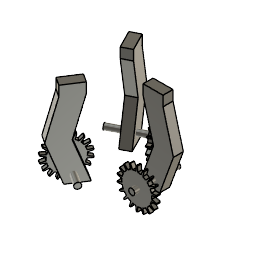
assembly_without_electronics (Autodesk Fusion 360 archive; units mm, degrees)
design "Fingers"
part number: 2026-03-20-16-49-33-089
Autodesk Fusion 360 part; units mm, degrees
sketch "Sketch2" plane through (0, 0, 0) normal (0, 0, 1) x (1, 0, 0)
  circle A0 centre (-139.7, 25.4) radius 19.05
  line L0 (-140.9543, 44.4087) -> (-140.4015, 50.7345)
  line L1 (-138.4228, 44.4071) -> (-138.9798, 50.7327)
  line L2 (-140.4015, 50.7345) -> (-138.9798, 50.7327)
  line L3 (-145.0006, 43.6977) -> (-147.6875, 49.4512)
  line L4 (-149.0241, 48.9668) -> (-147.6875, 49.4512)
  line L5 (-147.38, 42.8333) -> (-149.0241, 48.9668)
  line L6 (-150.9392, 40.7813) -> (-155.4318, 45.2689)
  line L7 (-156.5221, 44.3565) -> (-155.4318, 45.2689)
  line L8 (-152.8794, 39.1552) -> (-156.5221, 44.3565)
  line L9 (-155.5221, 36.0097) -> (-161.2786, 38.69)
  line L10 (-161.9911, 37.4598) -> (-161.2786, 38.69)
  line L11 (-156.7891, 33.8181) -> (-161.9911, 37.4598)
  line L12 (-158.1966, 29.9584) -> (-164.5227, 30.5082)
  line L13 (-164.7715, 29.1085) -> (-164.5227, 30.5082)
  line L14 (-158.6377, 27.4656) -> (-164.7715, 29.1085)
  line L15 (-158.6402, 23.3572) -> (-164.7729, 21.7103)
  line L16 (-164.5279, 20.3099) -> (-164.7729, 21.7103)
  line L17 (-158.2021, 20.8639) -> (-164.5279, 20.3099)
  line L18 (-156.7993, 17.0025) -> (-161.9988, 13.3574)
  line L19 (-161.2896, 12.1252) -> (-161.9988, 13.3574)
  line L20 (-155.5348, 14.8094) -> (-161.2896, 12.1252)
  line L21 (-152.896, 11.6607) -> (-156.5352, 6.457)
  line L22 (-155.4474, 5.5417) -> (-156.5352, 6.457)
  line L23 (-150.9577, 10.0323) -> (-155.4474, 5.5417)
  line L24 (-147.401, 7.976) -> (-149.041, 1.8414)
  line L25 (-147.7058, 1.3534) -> (-149.041, 1.8414)
  line L26 (-145.0227, 7.1087) -> (-147.7058, 1.3534)
  line L27 (-140.9772, 6.3929) -> (-140.4202, 0.0673)
  line L28 (-138.9985, 0.0655) -> (-140.4202, 0.0673)
  line L29 (-138.4457, 6.3913) -> (-138.9985, 0.0655)
  line L30 (-134.3994, 7.1023) -> (-131.7125, 1.3488)
  line L31 (-130.3759, 1.8332) -> (-131.7125, 1.3488)
  line L32 (-132.02, 7.9667) -> (-130.3759, 1.8332)
  line L33 (-128.4608, 10.0187) -> (-123.9682, 5.5311)
  line L34 (-122.8779, 6.4435) -> (-123.9682, 5.5311)
  line L35 (-126.5206, 11.6448) -> (-122.8779, 6.4435)
  line L36 (-123.8779, 14.7903) -> (-118.1214, 12.11)
  line L37 (-117.4089, 13.3402) -> (-118.1214, 12.11)
  line L38 (-122.6109, 16.9819) -> (-117.4089, 13.3402)
  line L39 (-121.2034, 20.8416) -> (-114.8773, 20.2918)
  line L40 (-114.6285, 21.6915) -> (-114.8773, 20.2918)
  line L41 (-120.7623, 23.3344) -> (-114.6285, 21.6915)
  line L42 (-120.7598, 27.4428) -> (-114.6272, 29.0897)
  line L43 (-114.8722, 30.4901) -> (-114.6272, 29.0897)
  line L44 (-121.1979, 29.9361) -> (-114.8722, 30.4901)
  line L45 (-122.6007, 33.7975) -> (-117.4012, 37.4426)
  line L46 (-118.1104, 38.6748) -> (-117.4012, 37.4426)
  line L47 (-123.8652, 35.9906) -> (-118.1104, 38.6748)
  line L48 (-126.5041, 39.1393) -> (-122.8648, 44.343)
  line L49 (-123.9526, 45.2583) -> (-122.8648, 44.343)
  line L50 (-128.4423, 40.7677) -> (-123.9526, 45.2583)
  line L51 (-131.999, 42.824) -> (-130.359, 48.9586)
  line L52 (-131.6942, 49.4466) -> (-130.359, 48.9586)
  line L53 (-134.3773, 43.6913) -> (-131.6942, 49.4466)
  dimension "d14" = 38.1
  dimension "d15" = 6.35
  dimension "d16" = 6.35
  dimension "d18" = 360
  constraint coincident A0 L0.start
  constraint coincident A0 L1.start
  measures "d14" diameter of A0
  measures "d15" distance of L0.start L0.end
  measures "d16" distance of L1.start L1.end
extrude "Extrude3" add sketch "Sketch2" along normal blind 5.08 makes body 1
sketch "Sketch3" plane through (0, 0, 0) normal (0, 0, 1) x (1, 0, 0)
  line L0 (0, 0) -> (17.3334, 47.7514)
  line L1 (-25.4, 0) -> (-7.9907, 47.7237)
  line L2 (17.3334, 47.7514) -> (4.2196, 96.8296)
  line L3 (-7.9907, 47.7237) -> (-21.1192, 96.798)
  line L4 (-21.1192, 96.798) -> (4.2196, 96.8296)
  line L5 (-25.4, 0) -> (0, 0)
  dimension "d21" = 50.8
  dimension "d22" = 50.8
  dimension "d23" = 50.8
  dimension "d24" = 50.8
  constraint coincident L0.start L5.end
  constraint horizontal L5
  measures "d21" distance of L0.start L0.end
  measures "d22" distance of L1.start L1.end
  measures "d23" distance of L0.end L2.end
  measures "d24" distance of L1.end L3.end
extrude "Extrude4" add sketch "Sketch3" along normal blind 12.7 separate body makes body 2
move_body "Move2" bodies 1 to x (1, 0, 0) y (0, 1, 0) z (0, 0, 1) at (130.81, -15.24, 12.7)
sketch "Sketch4" plane through (0, 0, 17.78) normal (0, 0, 1) x (-1, 0, 0)
  line L0 (7.6128, -29.1671) -> (8.1698, -35.4927)
  line L1 (8.1698, -35.4927) -> (9.5915, -35.4945)
  line L2 (9.5915, -35.4945) -> (10.1443, -29.1687)
  arc A0 (10.1443, -29.1687) -> (14.1906, -28.4577) centre (8.89, -10.16) ccw
  line L3 (14.1906, -28.4577) -> (16.8775, -34.2112)
  line L4 (16.8775, -34.2112) -> (18.2141, -33.7268)
  line L5 (18.2141, -33.7268) -> (16.57, -27.5933)
  arc A1 (16.57, -27.5933) -> (20.1292, -25.5413) centre (8.89, -10.16) ccw
  line L6 (20.1292, -25.5413) -> (24.6218, -30.0289)
  line L7 (24.6218, -30.0289) -> (25.7121, -29.1165)
  line L8 (25.7121, -29.1165) -> (22.0694, -23.9152)
  arc A2 (22.0694, -23.9152) -> (24.7121, -20.7697) centre (8.89, -10.16) ccw
  line L9 (24.7121, -20.7697) -> (30.4686, -23.45)
  line L10 (30.4686, -23.45) -> (31.1811, -22.2198)
  line L11 (31.1811, -22.2198) -> (25.9791, -18.5781)
  arc A3 (25.9791, -18.5781) -> (27.3866, -14.7184) centre (8.89, -10.16) ccw
  line L12 (27.3866, -14.7184) -> (33.7127, -15.2682)
  line L13 (33.7127, -15.2682) -> (33.9615, -13.8685)
  line L14 (33.9615, -13.8685) -> (27.8277, -12.2256)
  arc A4 (27.8277, -12.2256) -> (27.8302, -8.1172) centre (8.89, -10.16) ccw
  line L15 (27.8302, -8.1172) -> (33.9629, -6.4703)
  line L16 (33.9629, -6.4703) -> (33.7179, -5.0699)
  line L17 (33.7179, -5.0699) -> (27.3921, -5.6239)
  arc A5 (27.3921, -5.6239) -> (25.9893, -1.7625) centre (8.89, -10.16) ccw
  line L18 (25.9893, -1.7625) -> (31.1888, 1.8826)
  line L19 (31.1888, 1.8826) -> (30.4796, 3.1148)
  line L20 (30.4796, 3.1148) -> (24.7248, 0.4306)
  arc A6 (24.7248, 0.4306) -> (22.086, 3.5793) centre (8.89, -10.16) ccw
  line L21 (22.086, 3.5793) -> (25.7252, 8.783)
  line L22 (25.7252, 8.783) -> (24.6374, 9.6983)
  line L23 (24.6374, 9.6983) -> (20.1477, 5.2077)
  arc A7 (20.1477, 5.2077) -> (16.591, 7.264) centre (8.89, -10.16) ccw
  line L24 (16.591, 7.264) -> (18.231, 13.3986)
  line L25 (18.231, 13.3986) -> (16.8958, 13.8866)
  line L26 (16.8958, 13.8866) -> (14.2127, 8.1313)
  arc A8 (14.2127, 8.1313) -> (10.1672, 8.8471) centre (8.89, -10.16) ccw
  line L27 (10.1672, 8.8471) -> (9.6102, 15.1727)
  line L28 (9.6102, 15.1727) -> (8.1885, 15.1745)
  line L29 (8.1885, 15.1745) -> (7.6357, 8.8487)
  arc A9 (7.6357, 8.8487) -> (3.5894, 8.1377) centre (8.89, -10.16) ccw
  line L30 (3.5894, 8.1377) -> (0.9025, 13.8912)
  line L31 (0.9025, 13.8912) -> (-0.4341, 13.4068)
  line L32 (-0.4341, 13.4068) -> (1.21, 7.2733)
  arc A10 (1.21, 7.2733) -> (-2.3492, 5.2213) centre (8.89, -10.16) ccw
  line L33 (-2.3492, 5.2213) -> (-6.8418, 9.7089)
  line L34 (-6.8418, 9.7089) -> (-7.9321, 8.7965)
  line L35 (-7.9321, 8.7965) -> (-4.2894, 3.5952)
  arc A11 (-4.2894, 3.5952) -> (-6.9321, 0.4497) centre (8.89, -10.16) ccw
  line L36 (-6.9321, 0.4497) -> (-12.6886, 3.13)
  line L37 (-12.6886, 3.13) -> (-13.4011, 1.8998)
  line L38 (-13.4011, 1.8998) -> (-8.1991, -1.7419)
  arc A12 (-8.1991, -1.7419) -> (-9.6066, -5.6016) centre (8.89, -10.16) ccw
  line L39 (-9.6066, -5.6016) -> (-15.9327, -5.0518)
  line L40 (-15.9327, -5.0518) -> (-16.1815, -6.4515)
  line L41 (-16.1815, -6.4515) -> (-10.0477, -8.0944)
  arc A13 (-10.0477, -8.0944) -> (-10.0502, -12.2028) centre (8.89, -10.16) ccw
  line L42 (-10.0502, -12.2028) -> (-16.1828, -13.8497)
  line L43 (-16.1828, -13.8497) -> (-15.9378, -15.2501)
  line L44 (-15.9378, -15.2501) -> (-9.6121, -14.6961)
  arc A14 (-9.6121, -14.6961) -> (-8.2093, -18.5575) centre (8.89, -10.16) ccw
  line L45 (-8.2093, -18.5575) -> (-13.4088, -22.2026)
  line L46 (-13.4088, -22.2026) -> (-12.6996, -23.4348)
  line L47 (-12.6996, -23.4348) -> (-6.9448, -20.7506)
  arc A15 (-6.9448, -20.7506) -> (-4.3059, -23.8993) centre (8.89, -10.16) ccw
  line L48 (-4.3059, -23.8993) -> (-7.9452, -29.103)
  line L49 (-7.9452, -29.103) -> (-6.8574, -30.0183)
  line L50 (-6.8574, -30.0183) -> (-2.3677, -25.5277)
  arc A16 (-2.3677, -25.5277) -> (1.189, -27.584) centre (8.89, -10.16) ccw
  line L51 (1.189, -27.584) -> (-0.451, -33.7186)
  line L52 (-0.451, -33.7186) -> (0.8842, -34.2066)
  line L53 (0.8842, -34.2066) -> (3.5673, -28.4513)
  arc A17 (3.5673, -28.4513) -> (7.6128, -29.1671) centre (8.89, -10.16) ccw
  circle A18 centre (8.89, -10.16) radius 3.81
  dimension "d27" = 7.62
  constraint concentric A0 A18
  measures "d27" diameter of A18
extrude "Extrude5" add sketch "Sketch4" along normal mid plane 58.42 separate body contours A18 makes body 3
move_body "Move3" bodies 3 to x (1, 0, 0) y (0, 1, 0) z (0, 0, 1) at (0, 0, -7.62)
copy_body "CopyPasteBodies1" bodies 2 makes body 4
move_body "Move4" bodies 4 to x (1, 0, 0) y (0, 1, 0) z (0, 0, 1) at (-88.9, 0, 0)
copy_body "CopyPasteBodies2" bodies 3 makes body 5
move_body "Move5" bodies 5 to x (1, 0, 0) y (0, 1, 0) z (0, 0, 1) at (-88.9, 0, 0)
copy_body "CopyPasteBodies3" bodies 1 makes body 6
move_body "Move6" bodies 6 to x (1, 0, 0) y (0, 1, 0) z (0, 0, 1) at (-88.9, 0, 0)
copy_body "CopyPasteBodies4" bodies 4 6 5 makes body 7 makes body 8 makes body 9
move_body "Move7" bodies 7 8 9 to x (1, 0, 0) y (0, 1, 0) z (0, 0, 1) at (-88.9, 0, 0)
move_body "Move8" bodies 7 9 8 to x (1, 0, 0) y (0, 0, 1) z (0, -1, 0) at (0, 61.1148, -35.7148)
move_body "Move9" bodies 4 6 5 to x (1, 0, 0) y (0, 0, 1) z (0, -1, 0) at (0, 61.1148, -35.7148)
move_body "Move10" bodies 2 1 3 to x (1, 0, 0) y (0, 0, 1) z (0, -1, 0) at (0, 61.1148, -35.7148)
move_body "Move12" bodies 7 9 8 to x (-0.499998, -0.866025, -0.001867) y (0.866025, -0.5, 0.001078) z (-0.001867, -0.001078, 0.999998) at (-232.0022, -105.7721, 54.0724)
move_body "Move13" bodies 2 3 1 to x (1, 0, 0) y (0, 1, 0) z (0, 0, 1) at (13.057, 0, 35.7928)
move_body "Move14" bodies 7 8 9 to x (1, 0, 0) y (0, 1, 0) z (0, 0, 1) at (0.0119, -0.0068, -12.7)
move_body "Move15" bodies 4 5 6 to x (-0.499998, 0.866025, -0.001867) y (-0.866025, -0.5, -0.001078) z (-0.001867, 0.001078, 0.999998) at (-79.3477, 216.7581, 35.0807)
move_body "Move16" bodies 7 9 8 to x (0.996195, 0.087156, -0.000005) y (-0.087156, 0.996195, -0.000108) z (-0.000005, 0.000108, 1) at (52.7816, -0.8822, 0.0657)
move_body "Move17" bodies 4 5 6 to x (1, 0, 0) y (0, 1, 0) z (0, 0, 1) at (35.5478, -23.4706, 0.0443)
move_body "Move18" bodies 7 9 8 to x (1, 0, 0) y (0, 1, 0) z (0, 0, 1) at (0, 6.35, 0)
move_body "Move19" bodies 7 9 8 to x (0.996195, -0.087156, -0.000005) y (0.087156, 0.996195, 0.000108) z (-0.000005, -0.000108, 1) at (-2.3742, -3.4539, -0.003)
move_body "Move20" bodies 7 8 9 to x (1, 0, 0) y (0, 1, 0) z (0, 0, 1) at (-5.08, -5.08, -0.0063)
move_body "Move21" bodies 7 8 9 to x (0.996195, 0.087156, -0.000005) y (-0.087156, 0.996195, -0.000108) z (-0.000005, 0.000108, 1) at (-3.4779, -1.0089, -0.0043)
move_body "Move22" bodies 7 8 9 to x (0.984808, -0.173648, -0.000019) y (0.173648, 0.984808, 0.000216) z (-0.000019, -0.000216, 1) at (-8.5106, -13.6864, -0.0106)
move_body "Move23" bodies 7 8 9 to x (1, 0, 0) y (0, 1, 0) z (0, 0, 1) at (-5.08, -5.08, -0.0063)
move_body "Move24" bodies 7 9 8 to x (1, 0, 0) y (0, 1, 0) z (0, 0, 1) at (2.54, 2.54, 0.0032)
move_body "Move25" bodies 7 8 9 to x (1, 0, 0) y (0, 1, 0) z (0, 0, 1) at (0.0053, -0.0037, -6.35)
move_body "Move26" bodies 4 5 6 to x (1, 0, 0) y (0, 1, 0) z (0, 0, 1) at (-20.32, 20.32, -0.0253)
move_body "Move27" bodies 4 5 6 to x (1, 0, 0) y (0, 1, 0) z (0, 0, 1) at (2.54, -5.08, 0.0032)
move_body "Move28" bodies 4 5 6 to x (1, 0, 0) y (0, 1, 0) z (0, 0, 1) at (-5.08, -5.08, -0.0063)
move_body "Move29" bodies 4 5 6 to x (0.99863, -0.052336, -0.000002) y (0.052336, 0.99863, 0.000065) z (-0.000002, -0.000065, 1) at (-4.8953, -3.2973, -0.0061)
move_body "Move30" bodies 4 5 6 to x (1, 0, 0) y (0, 1, 0) z (0, 0, 1) at (1.1152, -2.1872, -0.6512)
move_body "Move31" bodies 1 to x (1, 0, 0) y (0, 1, 0) z (0, 0, 1) at (0, -15.24, 0)
move_body "Move32" bodies 8 to x (1, 0, 0) y (0, 1, 0) z (0, 0, 1) at (-12.4839, 8.7413, -0.0155)
move_body "Move33" bodies 6 to x (1, 0, 0) y (0, 1, 0) z (0, 0, 1) at (13.5789, 6.9188, 0.0169)
extrude "Extrude6" add 1 faces at (0.3841, 52.6481, 96.8866) along direction (-0.001245, 0, 0.999999) blind 12.7 on bodies 2 bodies 2
extrude "Extrude7" add 1 faces at (-54.4878, 9.9242, 96.5742) along direction (-0.001245, 0, 0.999999) blind 12.7 on bodies 7 bodies 7
extrude "Extrude8" add 1 faces at (-60.6085, 86.8346, 95.6716) along direction (-0.001245, 0, 0.999999) blind 12.7 on bodies 4 bodies 4
move_body "Move34" bodies 7 9 8 to x (0.996195, 0.087156, -0.000005) y (-0.087156, 0.996195, -0.000108) z (-0.000005, 0.000108, 1) at (0.4466, 5.1299, 0.0006)
move_body "Move35" bodies 7 9 8 to x (0.99863, -0.052336, -0.000002) y (0.052336, 0.99863, 0.000065) z (-0.000002, -0.000065, 1) at (-0.4821, -3.0524, -0.0006)

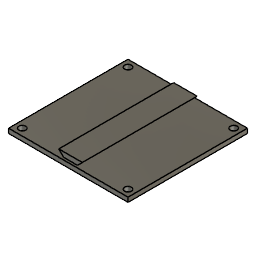
design "base_bottom"
part number: 2026-03-16-14-32-38-053
Autodesk Fusion 360 part; units mm, degrees
sketch "Sketch5" plane through (0, 0, 0) normal (0, 0, 1) x (1, 0, 0)
  line L0 (66.04, -66.04) -> (-66.04, -66.04)
  line L1 (-66.04, -66.04) -> (-66.04, 66.04)
  line L2 (-66.04, 66.04) -> (66.04, 66.04)
  line L3 (66.04, 66.04) -> (66.04, -66.04)
  line L4 (66.04, -66.04) -> (-66.04, 66.04) construction
  line L5 (-66.04, -66.04) -> (66.04, 66.04) construction
  constraint horizontal L0
  constraint perpendicular L0 L1
  constraint parallel L0 L2
  constraint parallel L1 L3
  constraint coincident L4 origin
  constraint coincident L5 origin
extrude "Extrude8" add sketch "Sketch5" along normal blind 5.08 makes body 1
sketch "Sketch6" plane through (0, 0, 5.08) normal (0, 0, 1) x (-1, 0, 0)
  line L0 (-66.04, -66.04) -> (66.04, -66.04)
  line L1 (66.04, -66.04) -> (66.04, 66.04)
  line L2 (66.04, 66.04) -> (-66.04, 66.04)
  line L3 (-66.04, 66.04) -> (-66.04, -66.04)
  circle A0 centre (58.42, -58.42) radius 3.81
  circle A1 centre (-58.42, -58.42) radius 3.81
  circle A2 centre (58.42, 58.42) radius 3.81
  circle A3 centre (-58.42, 58.42) radius 3.81
  dimension "d26" = 7.62
  dimension "d27" = 7.62
  dimension "d28" = 7.62
  dimension "d29" = 7.62
  measures "d26" diameter of A0
  measures "d27" diameter of A1
  measures "d28" diameter of A2
  measures "d29" diameter of A3
extrude "Extrude9" cut sketch "Sketch6" against normal blind 15.24 contours A0 | A1 | A2 | A3 bodies 1
sketch "Sketch7" plane through (0, 0, 5.08) normal (0, 0, 1) x (-1, 0, 0)
  circle A0 centre (58.42, -58.42) radius 3.81
  circle A1 centre (-58.42, -58.42) radius 3.81
  circle A2 centre (58.42, 58.42) radius 3.81
  circle A3 centre (-58.42, 58.42) radius 3.81
  line L0 (-66.04, -66.04) -> (66.04, -66.04)
  line L1 (66.04, -66.04) -> (66.04, 66.04)
  line L2 (66.04, 66.04) -> (-66.04, 66.04)
  line L3 (-66.04, 66.04) -> (-66.04, -66.04)
  circle A4 centre (0, 0) radius 62.8904
  dimension "d32" = 125.7808
  constraint coincident A4.centre origin
  measures "d32" diameter of A4
sketch "Sketch8" plane through (0, 0, 0) normal (0, 1, 0) x (1, 0, 0)
  line L0 (-7.62, -7.62) -> (-13.006, -13.0103)
  line L1 (7.62, -7.62) -> (13.0103, -13.006)
  line L2 (13.0103, -13.006) -> (-13.006, -13.0103)
  line L3 (7.62, -7.62) -> (-7.62, -7.62)
  dimension "d35" = 7.62
  dimension "d36" = 7.62
  constraint perpendicular L0 L1
  constraint horizontal L3
  measures "d35" distance of L0.start L0.end
  measures "d36" distance of L1.start L1.end
extrude "Extrude11" add sketch "Sketch8" along normal blind 63.5 and the other way blind 63.5 separate body makes body 2
move_body "Move1" bodies 2 to x (1, 0, 0) y (0, 1, 0) z (0, 0, 1) at (-0.0004, 0, -2.54)

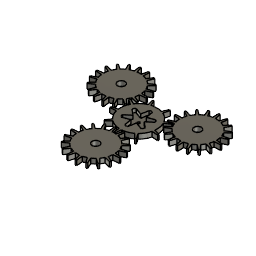
design "finger_gears" references "arm_middle"
part number: 2026-03-18-13-44-59-232
Autodesk Fusion 360 part; units mm, degrees
other "ExternalDerived1"
sketch "Sketch7" plane through (0, 0, 0) normal (0, 0, 1) x (1, 0, 0)
  circle A0 centre (0, 0) radius 19.05
  line L0 (1.2658, -19.0079) -> (0.716, -25.3341)
  line L1 (-1.3142, -19.0046) -> (-0.7583, -25.3302)
  line L2 (0.716, -25.3341) -> (-0.7583, -25.3302)
  line L3 (7.6905, -17.4287) -> (9.3375, -23.5613)
  line L4 (9.3375, -23.5613) -> (7.9509, -24.062)
  line L5 (5.265, -18.308) -> (7.9509, -24.062)
  line L6 (13.1877, -13.7473) -> (16.8329, -18.9468)
  line L7 (16.8329, -18.9468) -> (15.7011, -19.8915)
  line L8 (11.2092, -15.4031) -> (15.7011, -19.8915)
  line L9 (17.0942, -8.4078) -> (22.2979, -12.047)
  line L10 (22.2979, -12.047) -> (21.5575, -13.3218)
  line L11 (15.8014, -10.6405) -> (21.5575, -13.3218)
  line L12 (18.9389, -2.0541) -> (25.0735, -3.6941)
  line L13 (25.0735, -3.6941) -> (24.8137, -5.1453)
  line L14 (18.4877, -4.5944) -> (24.8137, -5.1453)
  line L15 (18.4993, 4.5472) -> (24.8248, 5.1043)
  line L16 (24.8248, 5.1043) -> (25.0771, 3.6518)
  line L17 (18.9441, 2.0059) -> (25.0771, 3.6518)
  line L18 (15.8284, 10.6001) -> (21.582, 13.2871)
  line L19 (21.582, 13.2871) -> (22.3158, 12.0084)
  line L20 (17.1156, 8.3642) -> (22.3158, 12.0084)
  line L21 (11.2484, 15.3745) -> (15.736, 19.8672)
  line L22 (15.736, 19.8672) -> (16.8628, 18.9167)
  line L23 (13.2227, 13.7136) -> (16.8628, 18.9167)
  line L24 (5.3116, 18.2945) -> (7.992, 24.0511)
  line L25 (7.992, 24.0511) -> (9.376, 23.5433)
  line L26 (7.7349, 17.409) -> (9.376, 23.5433)
  line L27 (-1.2658, 19.0079) -> (-0.716, 25.3341)
  line L28 (-0.716, 25.3341) -> (0.7583, 25.3302)
  line L29 (1.3142, 19.0046) -> (0.7583, 25.3302)
  line L30 (-7.6905, 17.4287) -> (-9.3375, 23.5613)
  line L31 (-9.3375, 23.5613) -> (-7.9509, 24.062)
  line L32 (-5.265, 18.308) -> (-7.9509, 24.062)
  line L33 (-13.1877, 13.7473) -> (-16.8329, 18.9468)
  line L34 (-16.8329, 18.9468) -> (-15.7011, 19.8915)
  line L35 (-11.2092, 15.4031) -> (-15.7011, 19.8915)
  line L36 (-17.0942, 8.4078) -> (-22.2979, 12.047)
  line L37 (-22.2979, 12.047) -> (-21.5575, 13.3218)
  line L38 (-15.8014, 10.6405) -> (-21.5575, 13.3218)
  line L39 (-18.9389, 2.0541) -> (-25.0735, 3.6941)
  line L40 (-25.0735, 3.6941) -> (-24.8137, 5.1453)
  line L41 (-18.4877, 4.5944) -> (-24.8137, 5.1453)
  line L42 (-18.4993, -4.5472) -> (-24.8248, -5.1043)
  line L43 (-24.8248, -5.1043) -> (-25.0771, -3.6518)
  line L44 (-18.9441, -2.0059) -> (-25.0771, -3.6518)
  line L45 (-15.8284, -10.6001) -> (-21.582, -13.2871)
  line L46 (-21.582, -13.2871) -> (-22.3158, -12.0084)
  line L47 (-17.1156, -8.3642) -> (-22.3158, -12.0084)
  line L48 (-11.2484, -15.3745) -> (-15.736, -19.8672)
  line L49 (-15.736, -19.8672) -> (-16.8628, -18.9167)
  line L50 (-13.2227, -13.7136) -> (-16.8628, -18.9167)
  line L51 (-5.3116, -18.2945) -> (-7.992, -24.0511)
  line L52 (-7.992, -24.0511) -> (-9.376, -23.5433)
  line L53 (-7.7349, -17.409) -> (-9.376, -23.5433)
  dimension "d61" = 38.1
  dimension "d62" = 6.35
  dimension "d63" = 6.35
  dimension "d65" = 360
  constraint coincident A0.centre origin
  constraint coincident A0 L0.start
  constraint coincident A0 L1.start
  measures "d61" diameter of A0
  measures "d62" distance of L0.start L0.end
  measures "d63" distance of L1.start L1.end
extrude "Extrude7" add sketch "Sketch7" along normal blind 5.08 makes body 1
copy_body "CopyPasteBodies1" bodies 1 makes body 2
move_body "Move19" bodies 2 to x (1, 0, 0) y (0, 1, 0) z (0, 0, 1) at (-60.96, 0, 0)
copy_body "CopyPasteBodies2" bodies 1 makes body 3
move_body "Move20" bodies 3 to x (1, 0, 0) y (0, 1, 0) z (0, 0, 1) at (73.66, 0, 0)
sketch "Sketch8" plane through (0, 0, 0) normal (0, 0, 1) x (1, 0, 0)
  circle A0 centre (0, 76.2) radius 19.05
  line L0 (1.2378, 57.1903) -> (0.685, 50.8644)
  line L1 (-1.2378, 57.1903) -> (-0.6861, 50.8643)
  line L2 (0.685, 50.8644) -> (-0.6861, 50.8643)
  line L3 (16.8102, 57.2321) -> (15.7599, 56.3507)
  line L4 (13.1674, 62.4333) -> (16.8102, 57.2321)
  line L5 (11.271, 60.842) -> (15.7599, 56.3507)
  line L6 (25.0697, 72.4751) -> (24.8317, 71.1248)
  line L7 (18.9359, 74.118) -> (25.0697, 72.4751)
  line L8 (18.506, 71.68) -> (24.8317, 71.1248)
  line L9 (21.5988, 89.4611) -> (22.2844, 88.2737)
  line L10 (15.844, 86.7769) -> (21.5988, 89.4611)
  line L11 (17.0818, 84.6329) -> (22.2844, 88.2737)
  line L12 (8.0216, 100.242) -> (9.31, 99.7731)
  line L13 (5.3385, 94.4867) -> (8.0216, 100.242)
  line L14 (7.6649, 93.64) -> (9.31, 99.7731)
  line L15 (-9.309, 99.7734) -> (-8.0206, 100.2425)
  line L16 (-7.6649, 93.64) -> (-9.309, 99.7734)
  line L17 (-5.3385, 94.4867) -> (-8.0206, 100.2425)
  line L18 (-22.2838, 88.2746) -> (-21.5983, 89.462)
  line L19 (-17.0818, 84.6329) -> (-22.2838, 88.2746)
  line L20 (-15.844, 86.7769) -> (-21.5983, 89.462)
  line L21 (-24.8318, 71.1259) -> (-25.07, 72.4762)
  line L22 (-18.506, 71.68) -> (-24.8318, 71.1259)
  line L23 (-18.9359, 74.118) -> (-25.07, 72.4762)
  line L24 (-15.7607, 56.3514) -> (-16.8111, 57.2327)
  line L25 (-11.271, 60.842) -> (-15.7607, 56.3514)
  line L26 (-13.1674, 62.4333) -> (-16.8111, 57.2327)
  dimension "d68" = 38.1
  dimension "d69" = 6.35
  dimension "d70" = 6.35
  dimension "d72" = 360
  constraint coincident A0 L0.start
  constraint coincident A0 L1.start
  measures "d68" diameter of A0
  measures "d69" distance of L0.start L0.end
  measures "d70" distance of L1.start L1.end
extrude "Extrude8" add sketch "Sketch8" along normal blind 5.08 separate body makes body 4
move_body "Move21" bodies 4 to x (1, 0, 0) y (0, 1, 0) z (0, 0, 1) at (43.18, -38.1, 0)
move_body "Move22" bodies 4 to x (1, 0, 0) y (0, 1, 0) z (0, 0, 1) at (-5.08, 0, 0)
move_body "Move23" bodies 4 to x (-1, 0, 0) y (0, 1, 0) z (0, 0, -1) at (76.2, 0, 7.62)
move_body "Move24" bodies 3 to x (0.990268, -0.139173, 0) y (0.139173, 0.990268, 0) z (0, 0, 1) at (3.1462, 72.4863, 0)
move_body "Move25" bodies 1 to x (0.999391, 0.034899, 0) y (-0.034899, 0.999391, 0) z (0, 0, 1) at (1.0397, 64.1158, 0.0186)
move_body "Move26" bodies 3 to x (0.965926, -0.258819, 0) y (0.258819, 0.965926, 0) z (0, 0, 1) at (-10.4016, 16.6906, 0.0245)
move_body "Move27" bodies 1 to x (0.939693, 0.34202, 0) y (-0.34202, 0.939693, 0) z (0, 0, 1) at (18.0551, -3.2469, 0.0176)
move_body "Move28" bodies 2 to x (0.984808, -0.173648, 0) y (0.173648, 0.984808, 0) z (0, 0, 1) at (98.3264, -16.9924, 91.5036)
sketch "Sketch13" plane through (0, 0, 96.5836) normal (0, 0, 1) x (-1, 0, 0)
  arc A0 (-24.5452, 19.5945) -> (-27.652, 22.2082) centre (-38.2925, 6.4068) ccw
  line L0 (-27.652, 22.2082) -> (-24.9707, 27.9643)
  line L1 (-24.9707, 27.9643) -> (-26.2455, 28.7047)
  line L2 (-26.2455, 28.7047) -> (-29.8847, 23.501)
  arc A1 (-29.8847, 23.501) -> (-33.6981, 24.8945) centre (-38.2925, 6.4068) ccw
  line L3 (-33.6981, 24.8945) -> (-33.1472, 31.2205)
  line L4 (-33.1472, 31.2205) -> (-34.5984, 31.4803)
  line L5 (-34.5984, 31.4803) -> (-36.2383, 25.3457)
  arc A2 (-36.2383, 25.3457) -> (-40.2983, 25.3509) centre (-38.2925, 6.4068) ccw
  line L6 (-40.2983, 25.3509) -> (-41.9443, 31.4839)
  line L7 (-41.9443, 31.4839) -> (-43.3968, 31.2317)
  line L8 (-43.3968, 31.2317) -> (-42.8397, 24.9061)
  arc A3 (-42.8397, 24.9061) -> (-46.6566, 23.5224) centre (-38.2925, 6.4068) ccw
  line L9 (-46.6566, 23.5224) -> (-50.3009, 28.7226)
  line L10 (-50.3009, 28.7226) -> (-51.5796, 27.9888)
  line L11 (-51.5796, 27.9888) -> (-48.8926, 22.2353)
  arc A4 (-48.8926, 22.2353) -> (-52.0061, 19.6295) centre (-38.2925, 6.4068) ccw
  line L12 (-52.0061, 19.6295) -> (-57.2091, 23.2697)
  line L13 (-57.2091, 23.2697) -> (-58.1597, 22.1428)
  line L14 (-58.1597, 22.1428) -> (-53.667, 17.6552)
  arc A5 (-53.667, 17.6552) -> (-55.7015, 14.1417) centre (-38.2925, 6.4068) ccw
  line L15 (-55.7015, 14.1417) -> (-61.8358, 15.7828)
  line L16 (-61.8358, 15.7828) -> (-62.3436, 14.3988)
  line L17 (-62.3436, 14.3988) -> (-56.587, 11.7185)
  arc A6 (-56.587, 11.7185) -> (-57.2971, 7.721) centre (-38.2925, 6.4068) ccw
  line L18 (-57.2971, 7.721) -> (-63.6227, 7.1651)
  line L19 (-63.6227, 7.1651) -> (-63.6265, 5.6908)
  line L20 (-63.6265, 5.6908) -> (-57.3004, 5.141)
  arc A7 (-57.3004, 5.141) -> (-56.6005, 1.1418) centre (-38.2925, 6.4068) ccw
  line L21 (-56.6005, 1.1418) -> (-62.3545, -1.5441)
  line L22 (-62.3545, -1.5441) -> (-61.8538, -2.9307)
  line L23 (-61.8538, -2.9307) -> (-55.7212, -1.2837)
  arc A8 (-55.7212, -1.2837) -> (-53.6956, -4.8024) centre (-38.2925, 6.4068) ccw
  line L24 (-53.6956, -4.8024) -> (-58.184, -9.2943)
  line L25 (-58.184, -9.2943) -> (-57.2393, -10.4261)
  line L26 (-57.2393, -10.4261) -> (-52.0398, -6.7809)
  arc A9 (-52.0398, -6.7809) -> (-48.9329, -9.3946) centre (-38.2925, 6.4068) ccw
  line L27 (-48.9329, -9.3946) -> (-51.6143, -15.1507)
  line L28 (-51.6143, -15.1507) -> (-50.3395, -15.8911)
  line L29 (-50.3395, -15.8911) -> (-46.7002, -10.6874)
  arc A10 (-46.7002, -10.6874) -> (-42.8869, -12.0809) centre (-38.2925, 6.4068) ccw
  line L30 (-42.8869, -12.0809) -> (-43.4378, -18.4069)
  line L31 (-43.4378, -18.4069) -> (-41.9866, -18.6667)
  line L32 (-41.9866, -18.6667) -> (-40.3466, -12.5321)
  arc A11 (-40.3466, -12.5321) -> (-36.2866, -12.5373) centre (-38.2925, 6.4068) ccw
  line L33 (-36.2866, -12.5373) -> (-34.6407, -18.6703)
  line L34 (-34.6407, -18.6703) -> (-33.1882, -18.418)
  line L35 (-33.1882, -18.418) -> (-33.7453, -12.0925)
  arc A12 (-33.7453, -12.0925) -> (-29.9283, -10.7088) centre (-38.2925, 6.4068) ccw
  line L36 (-29.9283, -10.7088) -> (-26.2841, -15.909)
  line L37 (-26.2841, -15.909) -> (-25.0054, -15.1751)
  line L38 (-25.0054, -15.1751) -> (-27.6923, -9.4216)
  arc A13 (-27.6923, -9.4216) -> (-24.5789, -6.8159) centre (-38.2925, 6.4068) ccw
  line L39 (-24.5789, -6.8159) -> (-19.3758, -10.456)
  line L40 (-19.3758, -10.456) -> (-18.4253, -9.3291)
  line L41 (-18.4253, -9.3291) -> (-22.918, -4.8416)
  arc A14 (-22.918, -4.8416) -> (-20.8835, -1.3281) centre (-38.2925, 6.4068) ccw
  line L42 (-20.8835, -1.3281) -> (-14.7492, -2.9692)
  line L43 (-14.7492, -2.9692) -> (-14.2414, -1.5852)
  line L44 (-14.2414, -1.5852) -> (-19.998, 1.0952)
  arc A15 (-19.998, 1.0952) -> (-19.2879, 5.0926) centre (-38.2925, 6.4068) ccw
  line L45 (-19.2879, 5.0926) -> (-12.9623, 5.6485)
  line L46 (-12.9623, 5.6485) -> (-12.9584, 7.1228)
  line L47 (-12.9584, 7.1228) -> (-19.2846, 7.6726)
  arc A16 (-19.2846, 7.6726) -> (-19.9845, 11.6718) centre (-38.2925, 6.4068) ccw
  line L48 (-19.9845, 11.6718) -> (-14.2305, 14.3577)
  line L49 (-14.2305, 14.3577) -> (-14.7311, 15.7444)
  line L50 (-14.7311, 15.7444) -> (-20.8638, 14.0973)
  arc A17 (-20.8638, 14.0973) -> (-22.8893, 17.616) centre (-38.2925, 6.4068) ccw
  line L51 (-22.8893, 17.616) -> (-18.401, 22.1079)
  line L52 (-18.401, 22.1079) -> (-19.3457, 23.2397)
  line L53 (-19.3457, 23.2397) -> (-24.5452, 19.5945)
  circle A18 centre (-38.2925, 6.4068) radius 3.81
  circle A19 centre (-78.74, -57.15) radius 3.81
  circle A20 centre (3.3176, -57.4165) radius 3.81
  dimension "d93" = 7.62
  dimension "d94" = 7.62
  dimension "d95" = 7.62
  constraint concentric A0 A18
  measures "d93" diameter of A18
  measures "d94" diameter of A19
  measures "d95" diameter of A20
move_body "Move29" bodies 2 to x (1, 0, 0) y (0, 1, 0) z (0, 0, 1) at (0, 0, -88.9)
move_body "Move30" bodies 4 to x (1, 0, 0) y (0, 1, 0) z (0, 0, 1) at (0, 0, -2.54)
move_body "Move31" bodies 2 to x (1, 0, 0) y (0, 1, 0) z (0, 0, 1) at (0, 0, -2.54)
extrude "Extrude11" cut sketch "Sketch13" along normal blind 0 and the other way blind 106.68 contours A18 | A19 | A20 bodies 1 2 3
move_body "Move32" bodies 3 to x (0.984808, -0.173648, 0) y (0.173648, 0.984808, 0) z (0, 0, 1) at (-6.403, 10.7814, -0.0115)
move_body "Move33" bodies 1 to x (0.984808, 0.173648, 0) y (-0.173648, 0.984808, 0) z (0, 0, 1) at (7.6575, -2.701, -0.0412)
move_body "Move34" bodies 3 to x (0.939693, 0.34202, 0) y (-0.34202, 0.939693, 0) z (0, 0, 1) at (20.3537, -18.1148, -0.6132)
move_body "Move35" bodies 1 to x (0.939693, -0.34202, 0) y (0.34202, 0.939693, 0) z (0, 0, 1) at (-15.237, 8.2986, 0.7936)
move_body "Move36" bodies 3 to x (1, 0, 0) y (0, 1, 0) z (0, 0, 1) at (-0.4992, -0.2703, -0.0433)
move_body "Move37" bodies 1 to x (1, 0, 0) y (0, 1, 0) z (0, 0, 1) at (0.2124, 0.0655, 0.0216)
sketch "Sketch14" plane through (0, 0, 0) normal (0, 0, -1) x (1, 0, 0)
  arc A0 (56.606, -33.58) -> (51.2674, -24.3333) centre (38.1, -38.1) ccw
  line L0 (51.2674, -24.3333) -> (54.9111, -19.1327)
  line L1 (54.9111, -19.1327) -> (53.8607, -18.2514)
  line L2 (53.8607, -18.2514) -> (49.371, -22.742)
  arc A1 (49.371, -22.742) -> (39.3378, -19.0903) centre (38.1, -38.1) ccw
  line L3 (39.3378, -19.0903) -> (38.7861, -12.7643)
  line L4 (38.7861, -12.7643) -> (37.415, -12.7644)
  line L5 (37.415, -12.7644) -> (36.8622, -19.0903)
  arc A2 (36.8622, -19.0903) -> (26.829, -22.742) centre (38.1, -38.1) ccw
  line L6 (26.829, -22.742) -> (22.3401, -18.2507)
  line L7 (22.3401, -18.2507) -> (21.2898, -19.1321)
  line L8 (21.2898, -19.1321) -> (24.9326, -24.3333)
  arc A3 (24.9326, -24.3333) -> (19.594, -33.58) centre (38.1, -38.1) ccw
  line L9 (19.594, -33.58) -> (13.2683, -33.0248)
  line L10 (13.2683, -33.0248) -> (13.0303, -34.3751)
  line L11 (13.0303, -34.3751) -> (19.1641, -36.018)
  arc A4 (19.1641, -36.018) -> (21.0182, -46.5329) centre (38.1, -38.1) ccw
  line L12 (21.0182, -46.5329) -> (15.8156, -50.1737)
  line L13 (15.8156, -50.1737) -> (16.5012, -51.3611)
  line L14 (16.5012, -51.3611) -> (22.256, -48.6769)
  arc A5 (22.256, -48.6769) -> (30.4351, -55.54) centre (38.1, -38.1) ccw
  line L15 (30.4351, -55.54) -> (28.79, -61.6731)
  line L16 (28.79, -61.6731) -> (30.0784, -62.142)
  line L17 (30.0784, -62.142) -> (32.7615, -56.3867)
  arc A6 (32.7615, -56.3867) -> (43.4385, -56.3867) centre (38.1, -38.1) ccw
  line L18 (43.4385, -56.3867) -> (46.1206, -62.1425)
  line L19 (46.1206, -62.1425) -> (47.409, -61.6734)
  line L20 (47.409, -61.6734) -> (45.7649, -55.54)
  arc A7 (45.7649, -55.54) -> (53.944, -48.6769) centre (38.1, -38.1) ccw
  line L21 (53.944, -48.6769) -> (59.6983, -51.362)
  line L22 (59.6983, -51.362) -> (60.3838, -50.1746)
  line L23 (60.3838, -50.1746) -> (55.1818, -46.5329)
  arc A8 (55.1818, -46.5329) -> (57.0359, -36.018) centre (38.1, -38.1) ccw
  line L24 (57.0359, -36.018) -> (63.17, -34.3762)
  line L25 (63.17, -34.3762) -> (62.9318, -33.0259)
  line L26 (62.9318, -33.0259) -> (56.606, -33.58)
  circle A9 centre (38.1, -38.1) radius 3.81
  line L27 (41.91, -38.1) -> (39.7016, -50.6065)
  line L28 (34.29, -38.1) -> (36.4922, -50.6076)
  arc A10 (36.4922, -50.6076) -> (39.7016, -50.6065) centre (38.0964, -49.1206) ccw
  line L29 (36.195, -41.3996) -> (48.128, -45.7462)
  arc A11 (48.128, -45.7462) -> (49.7318, -42.9662) centre (47.6423, -43.6134) ccw
  line L30 (40.005, -34.8004) -> (49.7318, -42.9662)
  line L31 (40.005, -41.3996) -> (49.7358, -33.2386)
  arc A12 (49.7358, -33.2386) -> (48.1302, -30.4597) centre (47.6459, -32.5928) ccw
  line L32 (36.195, -34.8004) -> (48.1302, -30.4597)
  line L33 (41.91, -38.1) -> (39.7078, -25.5924)
  arc A13 (39.7078, -25.5924) -> (36.4984, -25.5935) centre (38.1036, -27.0794) ccw
  line L34 (34.29, -38.1) -> (36.4984, -25.5935)
  line L35 (40.005, -34.8004) -> (28.072, -30.4538)
  arc A14 (28.072, -30.4538) -> (26.4682, -33.2338) centre (28.5577, -32.5866) ccw
  line L36 (36.195, -41.3996) -> (26.4682, -33.2338)
  line L37 (36.195, -34.8004) -> (26.4642, -42.9614)
  arc A15 (26.4642, -42.9614) -> (28.0698, -45.7403) centre (28.5541, -43.6072) ccw
  line L38 (40.005, -41.3996) -> (28.0698, -45.7403)
  dimension "d100" = 7.62
  dimension "d101" = 12.7
  dimension "d102" = 12.7
  dimension "d104" = 360
  constraint concentric A0 A9
  constraint coincident A9 L27.start
  constraint coincident A9 L28.start
  measures "d100" diameter of A9
  measures "d101" distance of L27.start L27.end
  measures "d102" distance of L28.start L28.end
extrude "Extrude12" cut sketch "Sketch14" along normal blind 0 and the other way blind 1.27 contours A9 L33 | A9 L27 L30 L31 L33 | A9 L27 | A9 L27 L28 L29 L30 L31 L32 L33 L34 L35 L36 L37 L38 | A9 L30 L33 | A9 L27 L31 | A9 L30 | A9 L30 L32 L33 L35 | L30 L31 A12 L32 L33 | A9 L27 L29 L31 L38 | A9 L31 | L27 L29 A11 L30 L31 | A9 L35 | L32 L33 A13 L34 L35 | A9 L38 | L27 L28 A10 L29 L38 | A9 L32 L35 | A9 L32 L34 L35 L37 | A9 L29 L38 | A9 L28 L29 L36 L38 | A9 L32 | L34 L35 A14 L36 L37 | A9 L29 | L28 L36 L37 A15 L38 | A9 L37 | A9 L34 L37 | A9 L28 L34 L36 L37 | A9 L36 | A9 L28 L36 | A9 L34 | A9 L28 bodies 4
sketch "Sketch15" plane through (0, 0, 1.27) normal (0, 0, -1) x (1, 0, 0)
  arc A0 (28.072, -30.4538) -> (26.4682, -33.2338) centre (28.5577, -32.5866) ccw
  line L0 (26.4682, -33.2338) -> (32.2627, -38.0983)
  line L1 (32.2627, -38.0983) -> (26.4642, -42.9614)
  arc A1 (26.4642, -42.9614) -> (28.0698, -45.7403) centre (28.5541, -43.6072) ccw
  line L2 (28.0698, -45.7403) -> (35.1799, -43.1544)
  line L3 (35.1799, -43.1544) -> (36.4922, -50.6076)
  arc A2 (36.4922, -50.6076) -> (39.7016, -50.6065) centre (38.0964, -49.1206) ccw
  line L4 (39.7016, -50.6065) -> (41.0172, -43.1561)
  line L5 (41.0172, -43.1561) -> (48.128, -45.7462)
  arc A3 (48.128, -45.7462) -> (49.7318, -42.9662) centre (47.6423, -43.6134) ccw
  line L6 (49.7318, -42.9662) -> (43.9373, -38.1017)
  line L7 (43.9373, -38.1017) -> (49.7358, -33.2386)
  arc A4 (49.7358, -33.2386) -> (48.1302, -30.4597) centre (47.6459, -32.5928) ccw
  line L8 (48.1302, -30.4597) -> (41.0201, -33.0456)
  line L9 (41.0201, -33.0456) -> (39.7078, -25.5924)
  arc A5 (39.7078, -25.5924) -> (36.4984, -25.5935) centre (38.1036, -27.0794) ccw
  line L10 (36.4984, -25.5935) -> (35.1828, -33.0439)
  line L11 (35.1828, -33.0439) -> (28.072, -30.4538)
  circle A6 centre (38.1, -38.1) radius 1.27
  dimension "d109" = 2.54
  measures "d109" diameter of A6
extrude "Extrude13" cut sketch "Sketch15" along normal blind 0 and the other way blind 1.27 contours A6 bodies 4
move_body "Move38" bodies 1 to x (1, 0, 0) y (0, 1, 0) z (0, 0, 1) at (0, 0, -0.762)
extrude "Extrude14" cut 1 faces at (31.8375, 42.331, 1.27) along direction (0, 0, -1) blind 0 and the other way blind 2.54 on bodies 4 bodies 4
extrude "Extrude15" cut 1 faces at (37.9453, 37.7608, 2.54) along direction (0, 0, -1) blind 0 and the other way blind 1.27 on bodies 4 bodies 4
move_body "Move39" bodies 4 to x (-1, 0, 0) y (0, 1, 0) z (0, 0, -1) at (76.2003, 0, 5.08)
sketch "Sketch16" plane through (0, 0, 0) normal (0, 0, -1) x (1, 0, 0)
  arc A0 (24.9328, -24.3333) -> (19.5943, -33.58) centre (38.1003, -38.1) ccw
  line L0 (19.5943, -33.58) -> (13.2685, -33.0259)
  line L1 (13.2685, -33.0259) -> (13.0303, -34.3762)
  line L2 (13.0303, -34.3762) -> (19.1644, -36.018)
  arc A1 (19.1644, -36.018) -> (21.0184, -46.5329) centre (38.1003, -38.1) ccw
  line L3 (21.0184, -46.5329) -> (15.8164, -50.1746)
  line L4 (15.8164, -50.1746) -> (16.5019, -51.362)
  line L5 (16.5019, -51.362) -> (22.2563, -48.6769)
  arc A2 (22.2563, -48.6769) -> (30.4354, -55.54) centre (38.1003, -38.1) ccw
  line L6 (30.4354, -55.54) -> (28.7913, -61.6734)
  line L7 (28.7913, -61.6734) -> (30.0797, -62.1425)
  line L8 (30.0797, -62.1425) -> (32.7617, -56.3867)
  arc A3 (32.7617, -56.3867) -> (43.4388, -56.3867) centre (38.1003, -38.1) ccw
  line L9 (43.4388, -56.3867) -> (46.1218, -62.142)
  line L10 (46.1218, -62.142) -> (47.4103, -61.6731)
  line L11 (47.4103, -61.6731) -> (45.7652, -55.54)
  arc A4 (45.7652, -55.54) -> (53.9443, -48.6769) centre (38.1003, -38.1) ccw
  line L12 (53.9443, -48.6769) -> (59.6991, -51.3611)
  line L13 (59.6991, -51.3611) -> (60.3847, -50.1737)
  line L14 (60.3847, -50.1737) -> (55.1821, -46.5329)
  arc A5 (55.1821, -46.5329) -> (57.0362, -36.018) centre (38.1003, -38.1) ccw
  line L15 (57.0362, -36.018) -> (63.17, -34.3751)
  line L16 (63.17, -34.3751) -> (62.932, -33.0248)
  line L17 (62.932, -33.0248) -> (56.6063, -33.58)
  arc A6 (56.6063, -33.58) -> (51.2677, -24.3333) centre (38.1003, -38.1) ccw
  line L18 (51.2677, -24.3333) -> (54.9105, -19.1321)
  line L19 (54.9105, -19.1321) -> (53.8602, -18.2507)
  line L20 (53.8602, -18.2507) -> (49.3713, -22.742)
  arc A7 (49.3713, -22.742) -> (39.3381, -19.0903) centre (38.1003, -38.1) ccw
  line L21 (39.3381, -19.0903) -> (38.7853, -12.7644)
  line L22 (38.7853, -12.7644) -> (37.4142, -12.7643)
  line L23 (37.4142, -12.7643) -> (36.8625, -19.0903)
  arc A8 (36.8625, -19.0903) -> (26.8293, -22.742) centre (38.1003, -38.1) ccw
  line L24 (26.8293, -22.742) -> (22.3396, -18.2514)
  line L25 (22.3396, -18.2514) -> (21.2892, -19.1327)
  line L26 (21.2892, -19.1327) -> (24.9328, -24.3333)
  circle A9 centre (38.1003, -38.1) radius 1.27
  dimension "d122" = 2.54
  constraint concentric A0 A9
  measures "d122" diameter of A9
extrude "Extrude16" cut sketch "Sketch16" against normal blind 24.13 contours A9 bodies 4
